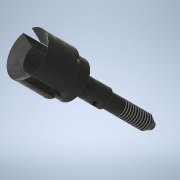
# Autodesk Inventor part: RCT-H005
Saved by Autodesk Inventor 2020 (Build 240168000, 168)
## iProperties
Created: 2019-01-29
Part Number: RCT-H005
Material: Generic
Document SubType Name: Modeling
Designer: Ehecatl Eli
Density: 1 g/cm^3
Appearance: Fine Textured - Black
Author: Ehecatl Eli
Autodesk Inventor part; units mm, degrees
ref_plane "YZ Plane" through (0, 0, 0) normal (1, 0, 0) x (0, 1, 0)
ref_plane "XZ Plane" through (0, 0, 0) normal (0, 1, 0) x (-1, 0, 0)
ref_plane "XY Plane" through (0, 0, 0) normal (0, 0, 1) x (1, 0, 0)
sketch "Sketch1" plane through (0, 0, 0) normal (1, 0, 0) x (0, 1, 0)
  line L0 (0, 0) -> (0, -9)
  line L1 (0, -9) -> (-1, -9)
  line L2 (-1, -9) -> (-1, -13)
  line L3 (-1, -13) -> (-3.5, -13)
  line L4 (-3.5, -13) -> (-3.5, -22)
  line L5 (-3.5, -22) -> (-4, -22)
  line L6 (-4, -22) -> (-4, -34)
  line L7 (-4, -34) -> (-5.1, -36)
  line L8 (-5.1, -36) -> (-6, -36)
  line L9 (0, 0) -> (-2.2, -2.5)
  line L10 (-2.2, -2.5) -> (-2.2, -9)
  line L11 (-6, -9.5) -> (-6, -36)
  line L12 (-2.2, -9) -> (-6, -9.5)
  dimension "d0" = 9
  dimension "d1" = 4
  dimension "d2" = 1
  dimension "d3" = 2.5
  dimension "d4" = 9
  dimension "d5" = 12
  dimension "d6" = 2
  dimension "d7" = 2
  dimension "d9" = 2.2
  dimension "d10" = 2.5
  dimension "d11" = 6.5
  dimension "d12" = 0.5
  dimension "d14" = 0.5
  dimension "d15" = 1.1
  constraints: 26 end point, 5 perpendicular, 3 parallel, 2 vertical, 1 coincident
  measures "d0" distance of L0.start L0.end
  measures "d1" distance of L1.end L2.end
  measures "d2" distance of L0.end L1.end
  measures "d3" distance of L2.end L3.end
  measures "d4" distance of L3.end L4.end
  measures "d5" distance of L5.end L6.end
  measures "d6" vertical distance of L7.end L6.end
  measures "d7" distance between parallel lines of L11 L6
  measures "d9" distance between parallel lines of L10 L0
  measures "d10" vertical distance of L9.end L0.start
  measures "d11" distance of L9.end L10.end
  measures "d12" vertical distance of L11.start L10.end
  measures "d14" distance of L4.end L5.end
  measures "d15" horizontal distance of L7.end L6.end
revolve "Revolution1" add sketch "Sketch1" angle 360 about axis through (0, -6, -9.5) along (0, 0, -1)
sketch "Sketch3" plane through (0, 0, 0) normal (1, 0, 0) x (0, 1, 0)
  line L0 (-4.75, 0) -> (-7.25, 0)
  line L1 (-7.25, 0) -> (-7.25, -10)
  line L2 (-4.75, -10) -> (-4.75, 0)
  arc A0 (-7.25, -10) -> (-4.75, -10) centre (-6, -10) ccw
  line L3 (0, -43.2) -> (0, 7.2) projected
  line L4 (-14.4, 0) -> (2.4, 0) projected
  point P0 (0, 0)
  dimension "d19" = 2.5
  dimension "d20" = 10
  dimension "d21" = 6
  constraints: 6 end point, 2 point on circle, 2 tangent, 1 centre point, 1 collinear, 1 horizontal, 1 parallel, 1 perpendicular
  measures "d19" distance of L0.start L0.end
  measures "d20" distance of L2.start L0.start
  measures "d21" distance from line of L3 A0.centre
extrude "Extrusion1" cut sketch "Sketch3" along normal through all both and the other way through all
sketch "Sketch4" plane through (0, 0, 0) normal (1, 0, 0) x (0, 1, 0)
  circle A0 centre (-6, -20) radius 1.1
  line L0 (0, -43.2) -> (0, 7.2) projected
  line L1 (-14.4, 0) -> (2.4, 0) projected
  point P0 (0, 0)
  dimension "d24" = 2.2
  dimension "d25" = 6
  dimension "d26" = 20
  constraints: 1 centre point
  measures "d24" diameter of A0
  measures "d25" distance from line of L0 A0.centre
  measures "d26" distance from line of L1 A0.centre
extrude "Extrusion2" cut sketch "Sketch4" along normal through all both and the other way through all
thread "Thread1" size "M4x0.7" class "6g" standard "ANSI Metric M Profile" length 8
body "Solid1"
